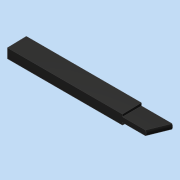
# Autodesk Inventor part: DivePlanesStabilizingFins_Print2
Saved by Autodesk Inventor 2017 (Build 210142000, 142)
## iProperties
Created: 2016-10-10
Part Number: DivePlanesStabilizingFins_Print2
Material: Generic
Document SubType Name: Modeling
Designer: techn
Density: 1 g/cm^3
Appearance: Glossy - Black
Author: techn
Autodesk Inventor part; units mm, degrees
ref_plane "YZ Plane" through (0, 0, 0) normal (1, 0, 0) x (0, 1, 0)
ref_plane "XZ Plane" through (0, 0, 0) normal (0, 1, 0) x (-1, 0, 0)
sketch "Sketch2" plane through (0, 0, 0) normal (0, 0, 1) x (1, 0, 0)
  line L0 (0, 0) -> (25.4, 0)
  line L1 (25.4, 0) -> (25.4, 5.588)
  line L2 (25.4, 5.588) -> (0, 5.588)
  line L3 (0, 5.588) -> (0, 0)
  arc A0 (25.4, 0) -> (25.4, 5.588) centre (25.4, 2.794) ccw
  dimension "d0" = 25.4
  dimension "d1" = 5.588
  constraints: 8 end point, 2 parallel, 2 point on circle, 2 tangent, 1 centre point, 1 horizontal, 1 perpendicular
  measures "d0" distance of L2.end L1.end
  measures "d1" distance of L1.end L0.end
ref_plane "Work Plane1" through (0, 0, 50.8) normal (0, 0, 1) x (1, 0, 0)
sketch "Sketch3" plane through (0, 0, 50.8) normal (0, 0, 1) x (1, 0, 0)
  line L0 (0, 1.2065) -> (6.35, 1.2065)
  line L1 (6.35, 1.2065) -> (6.35, 4.3815)
  line L2 (6.35, 4.3815) -> (0, 4.3815)
  line L3 (0, 4.3815) -> (0, 1.2065)
  arc A0 (6.35, 1.2065) -> (6.35, 4.3815) centre (6.35, 2.794) ccw
  point P0 (0, 0)
  dimension "d3" = 6.35
  dimension "d4" = 3.175
  dimension "d5" = 1.2065
  constraints: 8 end point, 2 parallel, 2 point on circle, 2 tangent, 1 centre point, 1 horizontal, 1 perpendicular
  measures "d3" distance of L2.end L1.end
  measures "d4" distance of L1.end L0.end
  measures "d5" distance of L0.start point (0, 0)
loft "Loft1" add profiles "Sketch2", "Sketch3"
sketch "Sketch4" plane through (0, 0, 0) normal (-1, 0, 0) x (0, 0, 1)
  line L0 (0, 5.588) -> (0, 0) projected
  line L1 (0, 0) -> (50.8, 1.2065) projected
  line L2 (50.8, 4.3815) -> (50.8, 1.2065) projected
  line L3 (0, 5.588) -> (50.8, 4.3815) projected
  line L4 (0, 5.588) -> (50.8, 4.3815) projected
  line L5 (44.45, 4.5323) -> (44.45, 1.0557)
  line L6 (50.8, 1.2065) -> (0, 0) projected
  dimension "d10" = 6.35
  constraints: 2 end point, 2 point on line, 1 vertical
  measures "d10" distance between parallel lines of L2 L5
extrude "Extrusion1" add sketch "Sketch4" along normal blind 38.608 contours L3 L2 L1 L5
sketch "Sketch5" plane through (25.4, 5.588, 0) normal (0, 0, -1) x (-1, 0, 0)
  line L0 (25.4, 0) -> (25.4, -5.588) projected
  line L1 (0, 0) -> (25.4, 0) projected
  arc A0 (0, 0) -> (0, -5.588) centre (0, -2.794) ccw projected
  line L2 (25.4, -5.588) -> (0, -5.588) projected
  line L3 (25.4, 0) -> (25.4, -5.588) projected
  line L4 (25.4, 0) -> (36.1487, 0)
  line L5 (36.1487, 0) -> (36.1487, -5.5776)
  line L6 (36.1487, -5.5776) -> (25.4, -5.5776)
  line L7 (25.4, -5.5776) -> (25.4, 0)
  line L8 (-3.175, -0.1076) -> (-3.175, -7.007)
  line L9 (25.4, -5.588) -> (0, -5.588) projected
  constraints: 10 end point, 3 parallel, 1 horizontal, 1 perpendicular, 1 vertical
revolve "Revolution1" add sketch "Sketch5" angle 15 about axis through (28.575, 5.4804, 0) along (0, -1, 0)
sketch "Sketch7" plane through (-10.7487, 5.588, 0) normal (0, 1, 0) x (1, 0, 0)
  line L0 (0, 0) -> (10.7487, 0) projected
  line L1 (36.1487, 0) -> (10.7487, 0) projected
  arc A0 (36.2569, 0.8218) -> (36.1487, 0) centre (39.3237, 0) ccw projected
  line L2 (1.3399, 10.1777) -> (36.2569, 0.8218) projected
  arc A1 (1.3399, 10.1777) -> (0, 0) centre (39.3237, 0) ccw projected
  line L3 (10.7487, 0) -> (10.7487, -44.45) projected
  line L4 (10.7487, 0) -> (-2.0556, 0)
  line L5 (-2.0556, 0) -> (-2.0556, 10.6947)
  line L6 (-2.0556, 10.6947) -> (10.7487, 10.6947)
  line L7 (10.7487, 10.6947) -> (10.7487, 0)
  constraints: 8 end point, 2 parallel, 1 horizontal, 1 perpendicular
extrude "Extrusion2" cut sketch "Sketch7" against normal blind 38.1 contours A1 L2 L7 L0 | L4 L5 L6 L7 L2 A1
sketch "Sketch8" plane through (0, 0.0104, -7.6566) normal (0.258819, 0, -0.9659258) x (-0.9659258, 0, -0.258819)
  line L0 (-29.583, 2.7836) -> (-24.8205, 2.7836)
  line L1 (-24.8205, 2.7836) -> (-8.9455, 2.7836)
  circle A0 centre (-24.8205, 2.7836) radius 1.27
  circle A1 centre (-8.9455, 2.7836) radius 1.27
  line L2 (-26.408, -0.0104) -> (0, -0.0104) projected
  point P0 (-1.9817, -0.0104)
  point P1 (0, 0)
  dimension "d17" = 4.7625
  dimension "d18" = 15.875
  dimension "d19" = 2.54
  dimension "d20" = 2.54
  dimension "d23" = 2.794
  constraints: 4 end point, 2 centre point, 2 coincident, 1 horizontal, 1 point on line, 1 other
  measures "d17" distance of L0.start L0.end
  measures "d18" distance of L0.end L1.end
  measures "d19" diameter of A0
  measures "d20" diameter of A1
extrude "Extrusion4" cut sketch "Sketch8" against normal blind 12.7
sketch "Sketch9" plane through (0, 1.0557, 44.45) normal (-1, 0, 0) x (0, 0, 1)
  line L0 (6.35, 0.1508) -> (6.35, 3.3258) projected
  line L1 (6.35, 3.3258) -> (0, 3.4766) projected
  line L2 (0, 3.4766) -> (0, 0) projected
  line L3 (0, 0) -> (6.35, 0.1508) projected
  line L4 (6.35, 3.3258) -> (6.35, 0.1508) projected
  line L5 (6.35, 2.5638) -> (0, 2.5638)
  line L6 (0, 3.4766) -> (0, 0) projected
  line L7 (6.35, 0.9128) -> (0, 0.9128)
  line L8 (6.35, 2.5638) -> (6.35, 4.769)
  line L9 (6.35, 4.769) -> (-56.0869, 8.5681)
  line L10 (-56.0869, 8.5681) -> (-57.3905, -12.8563)
  line L11 (-57.3905, -12.8563) -> (6.35, -0.7759)
  line L12 (6.35, -0.7759) -> (6.35, 0.9128)
  line L13 (0, 0.9128) -> (0, 0) construction
  line L14 (0, 2.5638) -> (0, 3.4766) construction
  line L15 (0, 2.5638) -> (0, 0.9128)
  point P0 (-44.45, -1.0557)
  dimension "d26" = 1.651
  constraints: 20 end point, 5 collinear, 5 point on line, 3 perpendicular
  measures "d26" distance between parallel lines of L5 L7
extrude "Extrusion5" cut sketch "Sketch9" against normal through all contours L3 L2 L7 L0 | L12 L11 L10 L9 L8 L1 L2 L3 | L5 L2 L1 L0
body "Solid1"
